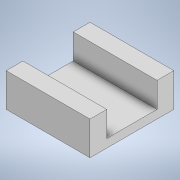
# Autodesk Inventor part: Тестовая коробка
Saved by Autodesk Inventor 2020 (Build 240168000, 168)
## iProperties
Created: 2021-04-26
Part Number: Тестовая коробка
Material: Типовые
Document SubType Name: Modeling
Designer: Антон
Density: 1 g/cm^3
Appearance: По умолчанию
Author: Антон
Autodesk Inventor part; units mm, degrees
ref_plane "YZ Plane" through (0, 0, 0) normal (1, 0, 0) x (0, 1, 0)
ref_plane "XZ Plane" through (0, 0, 0) normal (0, 1, 0) x (-1, 0, 0)
ref_plane "XY Plane" through (0, 0, 0) normal (0, 0, 1) x (1, 0, 0)
sketch "Эскиз1" plane through (0, 0, 0) normal (0, 1, 0) x (-1, 0, 0)
  line L0 (0, 0) -> (10, 0)
  line L1 (10, 0) -> (10, -10)
  line L2 (10, -10) -> (0, -10)
  line L3 (0, -10) -> (0, 0)
  dimension "d0" = 10
  dimension "d1" = 10
  constraints: 8 end point, 2 parallel, 1 horizontal, 1 perpendicular
  measures "d0" distance of L1.end L2.end
  measures "d1" distance of L0.end L1.end
extrude "Выдавливание1" add sketch "Эскиз1" along normal blind 4
sketch "Эскиз2" plane through (0, 4, 0) normal (0, 1, 0) x (1, 0, 0)
  line L0 (-10, 10) -> (-10, 0) projected
  line L1 (-10, 0) -> (-10, 2)
  line L2 (0, 0) -> (0, 10) projected
  line L3 (-10, 2) -> (0, 2)
  line L4 (0, 2) -> (0, 8)
  line L5 (0, 8) -> (-10, 8)
  line L6 (-10, 8) -> (-10, 2)
  line L7 (-10, 8) -> (-10, 10)
  line L8 (-10, 0) -> (0, 0) projected
  point P0 (0, 2)
  dimension "d4" = 2
  constraints: 12 end point, 2 collinear, 2 parallel, 2 point on line, 1 horizontal, 1 perpendicular
  measures "d4" distance between parallel lines of L8 L3
extrude "Выдавливание2" cut sketch "Эскиз2" against normal blind 3 contours L5 L2 L3 L0
